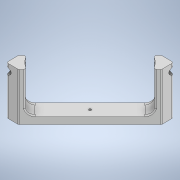
# Autodesk Inventor part: rotor_core
Saved by Autodesk Inventor 2021 (Build 250183000, 183)
## iProperties
Created: 2022-02-28
Part Number: rotor_core
Material: Generic
Document SubType Name: Modeling
Designer: ermoz
Density: 1 g/cm^3
Appearance: Default
Author: ermoz
Autodesk Inventor part; units mm, degrees
ref_plane "YZ Plane" through (0, 0, 0) normal (1, 0, 0) x (0, 1, 0)
ref_plane "XZ Plane" through (0, 0, 0) normal (0, 1, 0) x (-1, 0, 0)
ref_plane "XY Plane" through (0, 0, 0) normal (0, 0, 1) x (1, 0, 0)
sketch "Sketch1" plane through (0, 0, 0) normal (0, 1, 0) x (-1, 0, 0)
  line L0 (-12.5, -12.5) -> (12.5, -12.5)
  line L1 (12.5, -12.5) -> (12.5, 12.5)
  line L2 (12.5, 12.5) -> (-12.5, 12.5)
  line L3 (-12.5, 12.5) -> (-12.5, -12.5)
  line L4 (-12.5, -12.5) -> (12.5, 12.5) construction
  line L5 (12.5, -12.5) -> (-12.5, 12.5) construction
  line L6 (12.25, 12.25) -> (12.25, -12.25)
  line L7 (12.25, -12.25) -> (-12.25, -12.25)
  line L8 (-12.25, -12.25) -> (-12.25, 12.25)
  line L9 (-12.25, 12.25) -> (12.25, 12.25)
  circle A0 centre (0, 0) radius 13.5
  line L10 (-10.4822, -14.0178) -> (14.0178, 10.4822)
  line L11 (14.0178, 10.4822) -> (10.4822, 14.0178)
  line L12 (10.4822, 14.0178) -> (-14.0178, -10.4822)
  line L13 (-14.0178, -10.4822) -> (-10.4822, -14.0178)
  line L14 (-10.4822, -14.0178) -> (10.4822, 14.0178) construction
  line L15 (14.0178, 10.4822) -> (-14.0178, -10.4822) construction
  point P0 (-11.1486, -7.6131)
  point P1 (-12.25, -8.7145)
  point P2 (-8.7145, -12.25)
  point P3 (-7.6131, -11.1486)
  point P4 (8.7145, 12.25)
  point P5 (7.6131, 11.1486)
  point P6 (11.1486, 7.6131)
  point P7 (12.25, 8.7145)
  dimension "d0" = 25
  dimension "d1" = 25
  dimension "d2" = 0.25
  dimension "d3" = 27
  dimension "d4" = 5
  constraints: 32 end point, 7 parallel, 4 midpoint, 3 perpendicular, 1 centre point, 1 coincident, 1 horizontal, 3 other
  measures "d0" distance of L2.end L1.end
  measures "d1" distance of L1.end L0.end
  measures "d2" distance between parallel lines of L1 L6
  measures "d3" diameter of A0
  measures "d4" distance of L11.end L10.end
extrude "Extrusion1" add sketch "Sketch1" along normal blind 14 contours L8 L12 A0 L10 L7 | A0 L12 L9 L6 L10
extrude "Extrusion2" add sketch "Sketch1" along normal blind 2 contours A0 L12 L10
sketch "Sketch2" plane through (0, 2, 0) normal (0, 1, 0) x (1, 0, 0)
  circle A0 centre (0, 0) radius 0.35
  dimension "d9" = 0.7
  constraints: 1 centre point, 1 coincident
  measures "d9" diameter of A0
extrude "Extrusion3" cut sketch "Sketch2" against normal up to surface (2 mm away)
fillet "Fillet1" radius 0.5 10 edges at (12.25, 7, -12.25) (12.25, 7, -8.7145) (11.1486, 8, -7.6131) (7.6131, 8, -11.1486) (8.7145, 7, -12.25) (-7.6131, 8, 11.1486) (-11.1486, 8, 7.6131) (-12.25, 7, 8.7145) (-12.25, 7, 12.25) (-8.7145, 7, 12.25)
fillet "Fillet2" radius 2 6 edges at (-11.1764, 2, 7.885) (-7.885, 2, 11.1764) (-9.5459, 2, 9.5459) (11.1764, 2, -7.885) (7.885, 2, -11.1764) (9.5459, 2, -9.5459)
ref_plane "Work Plane2" through (9.5459, 0, -9.5459) normal (0.7071068, 0, -0.7071068) x (0, 1, 0)
ref_plane "Work Plane1" through (1.7678, 2, 1.7678) normal (0.7071068, 0, -0.7071068) x (0, 1, 0)
sketch "Sketch3" plane through (9.5459, 0, -9.5459) normal (0.7071068, 0, -0.7071068) x (0, 1, 0)
  circle A0 centre (12, 0) radius 1
  line L0 (14, 1.9286) -> (14, -1.9286) projected
  point P0 (0, 0)
  point P1 (14, 0)
  dimension "d14" = 2
  dimension "d15" = 2
  constraints: 1 centre point, 1 horizontal alignment, 1 midpoint
  measures "d14" diameter of A0
  measures "d15" distance from line of L0 A0.centre
extrude "Extrusion4" cut sketch "Sketch3" along normal mid plane 1000
chamfer "Chamfer1" distance 0.75 angle 45 6 edges at (9.4626, 12.9931, -9.6286) (9.6286, 12.9931, -9.4626) (10.2268, 11.9989, -8.8126) (9.5459, 11, -9.5459) (8.8126, 12, -10.2268) (-9.54, 11, 9.5519)
body "Solid1"
